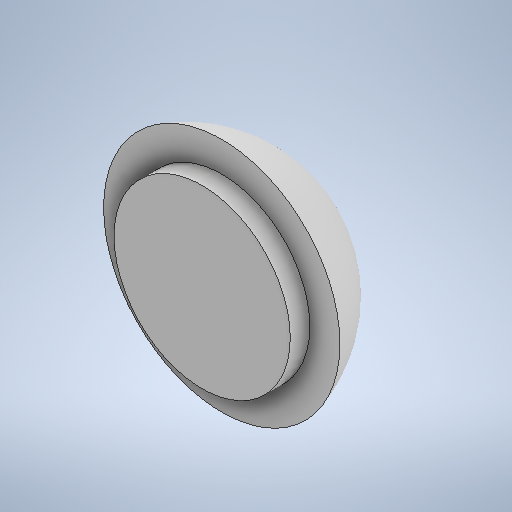
# Autodesk Inventor part: 140 cap
Saved by Autodesk Inventor 2025.1 (Build 291241000, 241)
## iProperties
Created: 2024-08-05
Part Number: 140 cap
Material: Generisch
Document SubType Name: Modeling
Designer: ffogue
Density: 1 g/cm^3
Appearance: Vorgabe
Author: ffogue
Autodesk Inventor part; units mm, degrees
ref_plane "YZ Plane" through (0, 0, 0) normal (1, 0, 0) x (0, 1, 0)
ref_plane "XZ Plane" through (0, 0, 0) normal (0, 1, 0) x (-1, 0, 0)
ref_plane "XY Plane" through (0, 0, 0) normal (0, 0, 1) x (1, 0, 0)
sketch "Sketch1" plane through (0, 0, 0) normal (0, 0, 1) x (1, 0, 0)
  line L0 (0, 0) -> (0, 5.5)
  arc A0 (6.0374, 1) -> (0, 5.5) centre (0, -0.8) ccw
  line L1 (6.0374, 1) -> (4.5, 1)
  line L2 (4.5, 1) -> (4.5, 0)
  line L3 (4.5, 0) -> (0, 0)
  dimension "d0" = 5.5
  dimension "d1" = 1
  dimension "d2" = 6.3
  dimension "d3" = 9
  constraints: 8 end point, 3 perpendicular, 2 point on circle, 1 centre point, 1 point on line, 1 vertical
  measures "d0" distance from line of L0.end L3
  measures "d1" distance of L1.end L2.end
  measures "d2" radius of A0
  measures "d3" diameter of L2 L0
revolve "Revolution1" add sketch "Sketch1" angle 360 about axis through (0, 0, 0) along (0, 1, 0)
body "Solid1"
